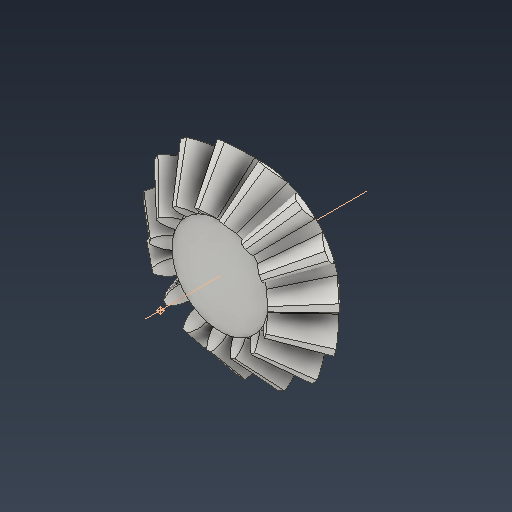
# Autodesk Inventor part: Коническая зубчатая передача1
Saved by Autodesk Inventor 2026 (Build 300175000, 175)
## iProperties
CustomPartVersion: 1
Created: 2026-01-11
Part Number: Коническая зубчатая передача1
Material: Steel, Mild
Document SubType Name: Modeling
Designer: GameHD
Categories: <?xml version="1.0" encoding="UTF-16"?> <MemberInstance><Categories><FamilyTemplate><FamilyTemplateParameter ValueType="xs:double" Id="1" ObjectReferenceKey="da_z" ObjectType="kUserParameterObject"/><FamilyTemplateParameter ValueType="xs:double" Id="2" ObjectReferenceKey="da_b" ObjectType="kUserParameterObject"/><FamilyTemplateParameter ValueType="xs:double" Id="3" ObjectReferenceKey="da_beta" ObjectType="kUserParameterObject"/><FamilyTemplateParameter ValueType="xs:double" Id="4" ObjectReferenceKey="da_dae" ObjectType="kUserParameterObject"/><FamilyTemplateParameter ValueType="xs:double" Id="5" ObjectReferenceKey="da_ve" ObjectType="kUserParameterObject"/><FamilyTemplateParameter ValueType="xs:double" Id="6" ObjectReferenceKey="da_omega" ObjectType="kUserParameterObject"/><FamilyTemplateParameter ValueType="xs:string" Id="7" ObjectReferenceKey="EAIAABAAAAAAHwAAAAAAAIAAAAAAAAAA" ObjectType="83914240" SubObjectId="SurfaceGeometry"/></FamilyTemplate><ParamToTemplateMap><ParamToTemplate CategoryParameter="//CategoryParameter[@InternalName='046C89C9-8512-4d59-83FE-43B91F4F132A']" TemplateParameter="1"/><ParamToTemplate CategoryParameter="//CategoryParameter[@InternalName='2552DF32-E462-4b46-AEBF-C6C7768E72AC']" TemplateParameter="2"/><ParamToTemplate CategoryParameter="//CategoryParameter[@InternalName='C9EE641D-15FC-4fae-A226-E94C4372FDD7']" TemplateParameter="3"/><ParamToTemplate><ParamToTemplate CategoryParameter="//CategoryParameter[@InternalName='00B6519A-459B-49c7-AD84-2E56D39A5744']" ConstantValue="0.000000"/></ParamToTemplate><ParamToTemplate><ParamToTemplate CategoryParameter="//CategoryParameter[@InternalName='04B31F0E-C7A6-4894-AA32-9629BEFACF47']" ConstantValue="1.000000"/></ParamToTemplate><ParamToTemplate><ParamToTemplate CategoryParameter="//CategoryParameter[@InternalName='43CBEC2E-7847-49e7-A936-2F7889FCB2D9']" ConstantValue="0.200000"/></ParamToTemplate><ParamToTemplate><ParamToTemplate CategoryParameter="//CategoryParameter[@InternalName='B1EFC894-105D-4ebd-86BF-FA20ED196853']" ConstantValue="0.300000"/></ParamToTemplate><ParamToTemplate><ParamToTemplate CategoryParameter="//CategoryParameter[@InternalName='51175063-3D10-4879-93E8-6246FE8B403D']" ConstantValue="2060000000.000000"/></ParamToTemplate><ParamToTemplate><ParamToTemplate CategoryParameter="//CategoryParameter[@InternalName='A3A52E27-4454-46a9-B0BD-C932399B70AF']" ConstantValue="0.300000"/></ParamToTemplate><ParamToTemplate CategoryParameter="//CategoryParameter[@InternalName='2A200944-5A8C-41ca-B96E-8520D2E510F1']" TemplateParameter="4"/><ParamToTemplate><ParamToTemplate CategoryParameter="//CategoryParameter[@InternalName='1A637F62-92C8-44bc-B81F-10802510B579']" ConstantValue="2.958880"/></ParamToTemplate><ParamToTemplate CategoryParameter="//CategoryParameter[@InternalName='B52DD4BE-6863-48fb-BF58-89EF6F9EC65C']" TemplateParameter="5"/><ParamToTemplate><ParamToTemplate CategoryParameter="//CategoryParameter[@InternalName='3956BFF2-84D2-457d-93C2-9B0613DEBA67']" ConstantValue="1.224509"/></ParamToTemplate><ParamToTemplate CategoryParameter="//CategoryParameter[@InternalName='739CFA02-461B-4bf8-8049-181FCAD8B28F']" TemplateParameter="6"/><ParamToTemplate><ParamToTemplate CategoryParameter="//CategoryParameter[@InternalName='A27E999F-E2CE-4481-8A2A-EBF499C4C3C5']" ConstantValue="0.000000"/></ParamToTemplate><ParamToTemplate><ParamToTemplate CategoryParameter="//CategoryParameter[@InternalName='9E1B4470-B2D3-4ff1-B813-535BB4CDF51A']" ConstantValue="3520000.000000"/></ParamToTemplate><ParamToTemplate><ParamToTemplate CategoryParameter="//CategoryParameter[@InternalName='F8452263-BFF6-458c-9FB1-07C4B99E95CD']" ConstantValue="11400000.000000"/></ParamToTemplate><ParamToTemplate><ParamToTemplate CategoryParameter="//CategoryParameter[@InternalName='3E3BB259-FD49-497f-8171-6EBC954A3479']" ConstantValue="2.000000"/></ParamToTemplate><ParamToTemplate CategoryParameter="//CategoryParameter[@InternalName='27C3BAF2-7550-4e4b-AE2C-0DB134B7D9B7']" TemplateParameter="7"/></ParamToTemplateMap><Category DisplayName="Gear" InternalName="DC85795E-93AB-48d5-8EEE-5A27447B64BD" Mnemonic="Gear"><CategoryParameter DisplayName="z" InternalName="046C89C9-8512-4d59-83FE-43B91F4F132A" Mnemonic="z"/><CategoryParameter DisplayName="b" InternalName="2552DF32-E462-4b46-AEBF-C6C7768E72AC" Mnemonic="b"/><CategoryParameter DisplayName="||b|" InternalName="C9EE641D-15FC-4fae-A226-E94C4372FDD7" Mnemonic="beta"/><CategoryParameter DisplayName="x" InternalName="00B6519A-459B-49c7-AD84-2E56D39A5744" Mnemonic="x"/><CategoryParameter DisplayName="a*" InternalName="04B31F0E-C7A6-4894-AA32-9629BEFACF47" Mnemonic="a"/><CategoryParameter DisplayName="c*" InternalName="43CBEC2E-7847-49e7-A936-2F7889FCB2D9" Mnemonic="c"/><CategoryParameter DisplayName="r|.f|*" InternalName="B1EFC894-105D-4ebd-86BF-FA20ED196853" Mnemonic="rf"/><CategoryParameter DisplayName="E" InternalName="51175063-3D10-4879-93E8-6246FE8B403D" Mnemonic="E"/><CategoryParameter DisplayName="||m|" InternalName="A3A52E27-4454-46a9-B0BD-C932399B70AF" Mnemonic="mi"/><Category DisplayName="BevelGear" InternalName="0C98F69A-0C2B-4791-B2FE-7691BB227E77" Mnemonic="BevelGear"><CategoryParameter DisplayName="d|.ae|" InternalName="2A200944-5A8C-41ca-B96E-8520D2E510F1" Mnemonic="dae"/><CategoryParameter DisplayName="d|.ai|" InternalName="1A637F62-92C8-44bc-B81F-10802510B579" Mnemonic="dai"/><CategoryParameter DisplayName="J|.e|" InternalName="B52DD4BE-6863-48fb-BF58-89EF6F9EC65C" Mnemonic="ve"/><CategoryParameter DisplayName="J|.i|" InternalName="3956BFF2-84D2-457d-93C2-9B0613DEBA67" Mnemonic="vi"/><CategoryParameter DisplayName="||S|" InternalName="739CFA02-461B-4bf8-8049-181FCAD8B28F" Mnemonic="omega"/><CategoryParameter DisplayName="x|.t|" InternalName="A27E999F-E2CE-4481-8A2A-EBF499C4C3C5" Mnemonic="xt"/><CategoryParameter DisplayName="||s||.Flim|" InternalName="9E1B4470-B2D3-4ff1-B813-535BB4CDF51A" Mnemonic="sFlim"/><CategoryParameter DisplayName="||s||.Hlim|" InternalName="F8452263-BFF6-458c-9FB1-07C4B99E95CD" Mnemonic="sHlim"/><CategoryParameter DisplayName="тип" InternalName="3E3BB259-FD49-497f-8171-6EBC954A3479" Mnemonic="type"/><CategoryParameter DisplayName="PitchDiameter" InternalName="27C3BAF2-7550-4e4b-AE2C-0DB134B7D9B7" Mnemonic="IDS_PITCHDIAM"/></Category></Category></Categories></MemberInstance>
Mass: 60.9118 g
Surface Area: 34.3074 cm^2
Volume: 7.7496 cm^3
Density: 7.86 g/cm^3
Appearance: Steel
Author: GameHD
Autodesk Inventor part; units mm, degrees
ref_plane "Плоскость сетки 2" through (0, 0, 0) normal (0.9781476, 0.2079117, 0) x (0, 0, 1)
sketch "Эскиз тела зубьев" plane through (0, 0, 0) normal (1, 0, 0) x (0, 1, 0)
  line L0 (0, 0) -> (19.954416, -25.045584) construction
  line L1 (19.954416, -25.045584) -> (24.62132, -20.37868)
  line L2 (24.62132, -20.37868) -> (0, 0) construction
  line L3 (22.5, -22.5) -> (0, 0) construction
  line L4 (11.990159, -15.049328) -> (14.794398, -12.24509)
  line L5 (19.954416, -25.045584) -> (11.990159, -15.049328)
  line L6 (24.62132, -20.37868) -> (14.794398, -12.24509)
  line L7 (0, -32.500143) -> (0, 5.41669)
  line L8 (0, -22.5) -> (24.62132, -22.5) construction
  dimension "d0" = 45
  dimension "d1" = 39.90883
  dimension "d2" = 49.24264
  dimension "d3" = 12.7
  dimension "d4" = 20.37868
  constraints: 16 end point, 4 point on line, 3 perpendicular, 2 collinear, 1 horizontal alignment, 1 vertical alignment
  measures "d0" diameter of L3.start L7
  measures "d1" diameter of L0.end L7
  measures "d2" diameter of L1.end L7
  measures "d3" distance between parallel lines of L1 L4
  measures "d4" vertical distance of L1.end L0.start
revolve "Тело зубьев" add sketch "Эскиз тела зубьев" angle 360 about axis through (0, 0, 0) along (0, 0, 1)
ref_plane "Плоскость зуба" through (0, 22.5, -22.5) normal (0, -0.7071068, 0.7071068) x (1, 0, 0)
sketch "Создать эскиз" plane through (0, 22.5, -22.5) normal (0, -0.7071068, 0.7071068) x (1, 0, 0)
  line L0 (0, -42.921075) -> (0, 12.513953)
  arc A0 (-1.28912, -4.392) -> (-6.113511, 4.468632) centre (-13.161798, -5.112679) ccw
  arc A1 (6.113511, 4.468632) -> (1.28912, -4.392) centre (13.161798, -5.112679) ccw
  line L1 (-1.28912, -4.392) -> (1.28912, -4.392)
  arc A2 (6.113511, 4.468632) -> (-6.113511, 4.468632) centre (0, -31.819805) ccw
  dimension "d7" = 11.89453
  dimension "d8" = 13.1618
  dimension "d9" = 26.70713
  dimension "d57" = 36.79981
  dimension "d58" = 27.42781
  constraints: 6 point on circle, 3 centre point, 3 symmetric about line, 2 end point, 1 coincident, 1 perpendicular, 1 other
  measures "d7" radius of A0
  measures "d8" horizontal distance of point (0, -31.82) A0.centre
  measures "d9" vertical distance of point (0, -31.82) A0.centre
  measures "d57" radius of A2
  measures "d58" distance from line of A2.centre L1
ref_plane "Конечная плоскость" through (0, 13.286399, -13.286399) normal (0, -0.7071068, 0.7071068) x (1, 0, 0)
sketch "Конечный эскиз" plane through (0, 13.286399, -13.286399) normal (0, -0.7071068, 0.7071068) x (1, 0, 0)
  line L0 (0, -32.249601) -> (0, 9.402606)
  arc A0 (-0.761234, -2.593505) -> (-3.610069, 2.638756) centre (-7.772129, -3.019071) ccw
  arc A1 (3.610069, 2.638756) -> (0.761234, -2.593505) centre (7.772129, -3.019071) ccw
  line L1 (-0.761234, -2.593505) -> (0.761234, -2.593505)
  arc A2 (3.610069, 2.638756) -> (-3.610069, 2.638756) centre (0, -18.789805) ccw
  dimension "d12" = 7.0238
  dimension "d15" = 7.77213
  dimension "d16" = 15.77073
  dimension "d59" = 21.73053
  dimension "d60" = 16.1963
  constraints: 6 point on circle, 3 centre point, 3 symmetric about line, 2 end point, 1 coincident, 1 other
  measures "d12" radius of A0
  measures "d15" horizontal distance of A0.centre point (0, -18.79)
  measures "d16" vertical distance of A0.centre point (0, -18.79)
  measures "d59" radius of A2
  measures "d60" distance from line of A2.centre L1
loft "Loft" cut profiles "Создать эскиз", "Конечный эскиз"
pattern_circular "Circular Pattern" count 15 over 360 about axis through (0, 0, 0) along (0, 0, 1) of "Loft"
sketch3d "3D эскиз: справа"
ref_plane "Конечная плоскость: справа" through (-0.169367, 13.285319, -13.286399) normal (0.0090137, -0.7070493, 0.7071068) x (0.9999187, 0.0127474, 0)
sketch "Конечный эскиз: справа" plane through (-0.169367, 13.285319, -13.286399) normal (0.0090137, -0.7070493, 0.7071068) x (0.9999187, 0.0127474, 0)
  arc A0 (-0.761234, -2.593505) -> (-3.610069, 2.638756) centre (-7.772129, -3.019071) ccw
  line L0 (0, -32.514526) -> (0, 9.667531)
  arc A1 (3.610069, 2.638756) -> (0.761234, -2.593505) centre (7.772129, -3.019071) ccw
  line L1 (-0.761234, -2.593505) -> (0.761234, -2.593505)
  arc A2 (3.610069, 2.638756) -> (-3.610069, 2.638756) centre (0, -18.789805) ccw
  dimension "d70" = 7.77213
  dimension "d71" = 15.77073
  dimension "d72" = 7.0238
  dimension "d73" = 16.1963
  dimension "d74" = 21.73053
  constraints: 6 point on circle, 3 centre point, 3 symmetric about line, 2 end point, 1 coincident, 1 perpendicular, 1 other
  measures "d70" horizontal distance of A2.centre A0.centre
  measures "d71" vertical distance of point (0, -18.79) A0.centre
  measures "d72" radius of A0
  measures "d73" distance from line of point (0, -18.79) L1
  measures "d74" radius of A2
feature "Лофт: справа" [suppressed]
pattern_circular "Круговой массив: справа" [suppressed]
sketch3d "3D эскиз: слева"
ref_plane "Конечная плоскость: cлева" through (0.153296, 13.285319, -13.286117) normal (-0.0081586, -0.707062, 0.7071045) x (0.9999334, -0.011538, 0)
sketch "Конечный эскиз: слева" plane through (0.153296, 13.285319, -13.286117) normal (-0.0081586, -0.707062, 0.7071045) x (0.9999334, -0.011538, 0)
  line L0 (0, -33.076001) -> (0, 9.926408)
  arc A0 (-0.761234, -2.593566) -> (-3.610069, 2.638695) centre (-7.772129, -3.019132) ccw
  arc A1 (3.610069, 2.638695) -> (0.761234, -2.593566) centre (7.772129, -3.019132) ccw
  line L1 (-0.761234, -2.593566) -> (0.761234, -2.593566)
  ellipse E0 centre (0, -8.658614) end of major axis (14.794398, -8.658614) minor radius 10.461185
  arc A2 (3.610069, 2.638695) -> (-3.610069, 2.638695) centre (0, -18.789866) ccw
  dimension "d56" = 10.46118
  dimension "d30" = 7.0238
  dimension "d31" = 7.77213
  dimension "d32" = 15.77073
  dimension "d61" = 21.73053
  dimension "d62" = 16.1963
  constraints: 6 point on circle, 3 centre point, 3 symmetric about line, 2 end point, 1 coincident, 2 other
  measures "d30" radius of A0
  measures "d31" horizontal distance of point (0, -18.79) A0.centre
  measures "d32" vertical distance of A0.centre point (0, -18.79)
  measures "d61" radius of A2
  measures "d62" distance from line of point (0, -18.79) L1
feature "Лофт: слева" [suppressed]
pattern_circular "Круговой массив: слева" [suppressed]
sketch "Эскиз тела" plane through (0, 0, 0) normal (1, 0, 0) x (0, 1, 0)
  line L0 (0, -28.383392) -> (0, -19.283816)
  line L1 (19.954416, -25.045584) -> (11.990159, -15.049328)
  line L2 (11.990159, -15.049328) -> (0, -15.049328)
  line L3 (19.954416, -25.045584) -> (0, -25.045584)
  constraints: 4 end point, 2 perpendicular, 2 point on line
sketch "Эскиз тела outline for Фиксировать тело" plane through (0, 0, 0) normal (1, 0, 0) x (0, 1, 0)
  line L0 (0, -25.045584) -> (19.954416, -25.045584)
  line L1 (0, -15.049328) -> (0, -25.045584)
  line L2 (11.990159, -15.049328) -> (0, -15.049328)
  line L3 (19.954416, -25.045584) -> (11.990159, -15.049328)
revolve "Фиксировать тело" add sketch "Эскиз тела outline for Фиксировать тело" angle 360 about axis through (0, 0, 0) along (0, 0, 1)
sketch "Sketch6" plane through (0, 0, 0) normal (1, 0, 0) x (0, 1, 0)
  line L0 (22.5, -22.5) -> (0, 0) projected
  line L1 (0, -29.7) -> (0, 4.95) projected
surface revolve "Средний диаметр" sketch "Sketch6" angle 360 about axis through (0, 0, 0) along (0, 0, 1) shown no curves L0
equation "\"d0\" = da_de"
equation "\"d1\" = da_dfe"
equation "\"d2\" = da_dae"
equation "\"d3\" = da_b"
equation "\"d4\" = da_ve"
equation "\"d7\" = fd_rr"
equation "\"d8\" = fd_x"
equation "\"d9\" = fd_y"
equation "\"d57\" = 0.5 * fd_dva + 0.3 * da_he"
equation "\"d58\" = 0.5 * fd_dva - 1.12 * da_he"
equation "\"da_teethtype\" = 0"
equation "\"da_b\" = 12.7"
equation "\"da_de\" = 45"
equation "\"da_dae\" = 49.24264"
equation "\"da_dfe\" = 39.90883"
equation "\"da_le\" = 31.81981"
equation "\"da_omega\" = 90deg"
equation "\"da_beta\" = 0"
equation "\"da_delta\" = 45deg"
equation "\"da_alpha\" = 20deg"
equation "\"da_he\" = 6.6"
equation "\"da_ve\" = 20.37868"
equation "\"da_zv\" = 21.213203"
equation "\"fd_loft\" = da_b + 0.05 * da_he"
equation "\"fd_x\" = fd_x1 + fd_x2"
equation "\"fd_y\" = fd_y1 - fd_y2"
equation "\"fd_dd\" = fd_dva - 0.8 * da_he"
equation "\"da_dvw\" = 63.63961"
equation "\"d11\" = fd_loft"
equation "\"da_dm\" = 36.01974"
equation "\"da_x\" = 0"
equation "\"da_m\" = 3"
equation "\"d50\" = da_omega"
equation "\"fd_rr\" = 11.894531"
equation "\"fd_dva\" = 69.63961"
equation "\"fd_x1\" = 2.380149"
equation "\"fd_x2\" = 10.781649"
equation "\"fd_y1\" = 31.730662"
equation "\"fd_y2\" = 5.023536"
body "Solid1"
body "Srf1"
